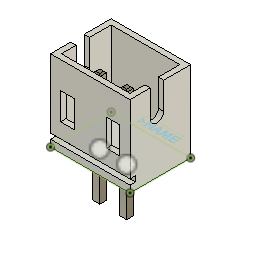
Connector-B2B-PH-K-S v3 (Autodesk Fusion 360 design; units mm, degrees)
Autodesk Fusion 360 part; units mm, degrees
sketch "Sketch1" plane through (0, 0, 0) normal (0, 0, 1) x (1, 0, 0)
  line L0 (-1.25, 0.25) -> (-0.75, 0.25)
  line L1 (-0.75, 0.25) -> (-0.75, -0.25)
  line L2 (-0.75, -0.25) -> (-1.25, -0.25)
  line L3 (-1.25, -0.25) -> (-1.25, 0.25)
  line L4 (0.75, 0.25) -> (1.25, 0.25)
  line L5 (1.25, 0.25) -> (1.25, -0.25)
  line L6 (1.25, -0.25) -> (0.75, -0.25)
  line L7 (0.75, -0.25) -> (0.75, 0.25)
  dimension "d1" = 0.5
  dimension "d2" = 0.5
  dimension "d3" = 0.5
  dimension "d4" = 0.5
  dimension "d5" = 0.75
  dimension "d6" = 0.75
  dimension "d7" = 0.25
  dimension "d8" = 0.25
  constraint horizontal L0
  constraint vertical L1
  constraint horizontal L2
  constraint vertical L3
  constraint horizontal L4
  constraint vertical L5
  constraint horizontal L6
  constraint vertical L7
  measures "d1" distance of L1 L3
  measures "d2" distance of L0 L2
  measures "d3" distance of L4.start L4.end
  measures "d4" distance of L4.end L5.end
  measures "d5" distance of origin L7
  measures "d6" distance of origin L1
  measures "d7" distance of origin L0
  measures "d8" distance of origin L4
extrude "Extrude1" add sketch "Sketch1" against normal blind 3.4 makes body 1 at (1.25, 0.0833, -1.1333) makes body 2 at (-1.0833, 0.25, -1.1333)
sketch "Sketch2" plane through (0, 0, 0) normal (0, 0, 1) x (1, 0, 0)
  line L0 (-2.95, 2.8) -> (2.95, 2.8)
  line L1 (2.95, 2.8) -> (2.95, -1.7)
  line L2 (2.95, -1.7) -> (-2.95, -1.7)
  line L3 (-2.95, -1.7) -> (-2.95, 2.8)
  dimension "d11" = 4.5
  dimension "d12" = 1.7
  dimension "d13" = 5.9
  dimension "d14" = 2.95
  constraint horizontal L0
  constraint vertical L1
  constraint horizontal L2
  constraint vertical L3
  measures "d11" distance of L0.start L2.end
  measures "d12" distance of origin L2
  measures "d13" distance of L1 L3
  measures "d14" distance of origin L1
extrude "Extrude2" add sketch "Sketch2" along normal blind 1 bodies 1 2
sketch "Sketch3" plane through (0, 0, 1) normal (0, 0, 1) x (-1, 0, 0)
  line L0 (2.95, 1.7) -> (-2.95, 1.7)
  line L1 (-2.95, 1.7) -> (-2.95, -2.8)
  line L2 (-2.95, -2.8) -> (2.95, -2.8)
  line L3 (2.95, -2.8) -> (2.95, 1.7)
  line L4 (2.55, 1.3) -> (-2.55, 1.3)
  line L5 (-2.55, 1.3) -> (-2.55, -2.4)
  line L6 (-2.55, -2.4) -> (2.55, -2.4)
  line L7 (2.55, -2.4) -> (2.55, 1.3)
  dimension "d17" = -0.4
extrude "Extrude3" add sketch "Sketch3" along normal blind 5 bodies 1
sketch "Sketch4" plane through (2.95, 0, 0) normal (1, 0, 0) x (0, 1, 0)
  line L0 (-1.7, 0) -> (2.8, 0)
  line L1 (2.8, 0) -> (2.8, 6)
  line L2 (2.8, 6) -> (-1.7, 6)
  line L3 (-1.7, 6) -> (-1.7, 0)
  line L4 (-0.2, 6) -> (-0.2, 4)
  line L5 (0.8, 6) -> (0.8, 4)
  arc A0 (-0.2, 4) -> (0.8, 4) centre (0.3, 4) ccw
  line L6 (-0.2, 6) -> (0.8, 6)
  dimension "d20" = 2
  dimension "d21" = 1.5
  dimension "d22" = 1
  dimension "d23" = 1
  dimension "d24" = 2
  constraint coincident L2 L4.start
  constraint perpendicular L2 L4
  constraint coincident L2 L5.start
  constraint perpendicular L2 L5
  measures "d20" distance of L3 A0.centre
  measures "d21" distance of L3 L4
  measures "d22" distance of L4 L5
  measures "d23" diameter of A0
  measures "d24" distance of L2 A0.centre
extrude "Extrude4" cut sketch "Sketch4" against normal blind 6 contours L2 L4 L5 A0 L6 bodies 1
sketch "Sketch5" plane through (0, -1.7, 0) normal (0, -1, 0) x (1, 0, 0)
  line L0 (-2.95, 0) -> (2.95, 0)
  line L1 (2.95, 0) -> (2.95, 6)
  line L2 (2.95, 6) -> (-2.95, 6)
  line L3 (-2.95, 6) -> (-2.95, 0)
  line L4 (-2.95, 0.9) -> (2.95, 0.9)
  line L5 (2.95, 0.9) -> (2.95, 0.5)
  line L6 (2.95, 0.5) -> (-2.95, 0.5)
  line L7 (-2.95, 0.5) -> (-2.95, 0.9)
  line L8 (-2.2, 4) -> (-1.2, 4)
  line L9 (-1.2, 4) -> (-1.2, 2)
  line L10 (-1.2, 2) -> (-2.2, 2)
  line L11 (-2.2, 2) -> (-2.2, 4)
  line L12 (1.2, 4) -> (2.2, 4)
  line L13 (2.2, 4) -> (2.2, 2)
  line L14 (2.2, 2) -> (1.2, 2)
  line L15 (1.2, 2) -> (1.2, 4)
  line L16 (-2.95, 0) -> (2.95, 0)
  dimension "d27" = 0.9
  dimension "d28" = 0.4
  dimension "d29" = 1
  dimension "d30" = 1
  dimension "d31" = 2
  dimension "d32" = 2
  dimension "d33" = 0.75
  dimension "d34" = 0.75
  dimension "d35" = 2
  dimension "d36" = 2
  constraint horizontal L4
  constraint vertical L5
  constraint horizontal L6
  constraint vertical L7
  constraint coincident L1 L5.end
  constraint coincident L3 L4.start
  constraint horizontal L8
  constraint vertical L9
  constraint horizontal L10
  constraint vertical L11
  constraint horizontal L12
  constraint vertical L13
  constraint horizontal L14
  constraint vertical L15
  measures "d27" distance of L4 L16
  measures "d28" distance of L4 L6
  measures "d29" distance of L8.start L8.end
  measures "d30" distance of L12.start L12.end
  measures "d31" distance of L12.start L14.end
  measures "d32" distance of L8.end L9.end
  measures "d33" distance of L3 L11
  measures "d34" distance of L1 L13
  measures "d35" distance of L2 L8
  measures "d36" distance of L2 L12
extrude "Extrude5" cut sketch "Sketch5" against normal blind 0.4 contours L1 L3 L4 L5 L6 L7 | L8 L9 L10 L11 | L12 L13 L14 L15 bodies 1
sketch "Sketch6" plane through (0, 0, 1) normal (0, 0, 1) x (-1, 0, 0)
  line L0 (2.55, 1.3) -> (-2.55, 1.3)
  line L1 (-2.55, 1.3) -> (-2.55, -2.4)
  line L2 (-2.55, -2.4) -> (2.55, -2.4)
  line L3 (2.55, -2.4) -> (2.55, 1.3)
  line L4 (0.75, 0.25) -> (1.25, 0.25)
  line L5 (1.25, 0.25) -> (1.25, -0.25)
  line L6 (1.25, -0.25) -> (0.75, -0.25)
  line L7 (0.75, -0.25) -> (0.75, 0.25)
  line L8 (-1.25, 0.25) -> (-0.75, 0.25)
  line L9 (-0.75, 0.25) -> (-0.75, -0.25)
  line L10 (-0.75, -0.25) -> (-1.25, -0.25)
  line L11 (-1.25, -0.25) -> (-1.25, 0.25)
extrude "Extrude6" add sketch "Sketch6" along normal blind 4 contours L4 L5 L6 L7 | L8 L9 L10 L11 bodies 1
chamfer "Chamfer1" distance 0.1 angle 45 16 edges at (1.25, 0, 5) (1, 0.25, 5) (0.75, 0, 5) (1, -0.25, 5) (-0.75, 0, 5) (-1, 0.25, 5) (-1.25, 0, 5) (-1, -0.25, 5) (1.25, 0, -3.4) (1, 0.25, -3.4) (0.75, 0, -3.4) (1, -0.25, -3.4) (-0.75, 0, -3.4) (-1, -0.25, -3.4) (-1.25, 0, -3.4) (-1, 0.25, -3.4) on bodies 1
equation "d14 = ( 5.9 / 2 ) * 1 mm"
